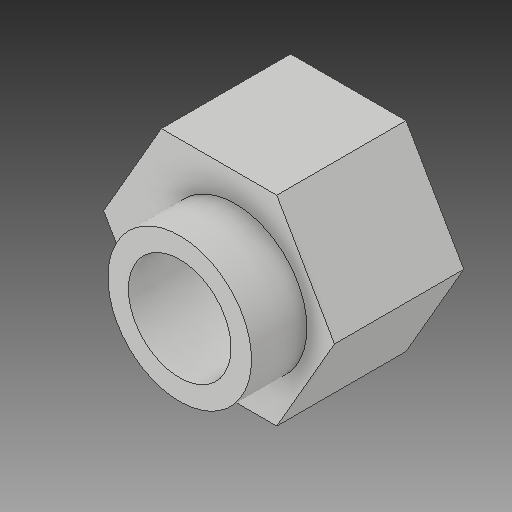
# Autodesk Inventor part: Eccentric Spacer
Saved by Autodesk Inventor 2018 (Build 220112000, 112)
## iProperties
Created: 2016-07-20
Part Number: Eccentric Spacer
Material: Generic
Document SubType Name: Modeling
Designer: User
Density: 1 g/cm^3
Appearance: Default
Mass: 0.445084 g
Surface Area: 5.38512 cm^2
Volume: 0.445084 cm^3
Author: User
Autodesk Inventor part; units mm, degrees
ref_plane "YZ Plane" through (0, 0, 0) normal (1, 0, 0) x (0, 1, 0)
ref_plane "XZ Plane" through (0, 0, 0) normal (0, 1, 0) x (-1, 0, 0)
ref_plane "XY Plane" through (0, 0, 0) normal (0, 0, 1) x (1, 0, 0)
sketch "Sketch1" plane through (0, 0, 0) normal (0, 0, 1) x (1, 0, 0)
  line L0 (-3.5818, 0) -> (-9.2068, 0)
  line L1 (-9.2068, 0) -> (-6.3943, 4.8714)
  line L2 (-6.3943, 4.8714) -> (-0.7693, 4.8714)
  line L3 (-0.7693, 4.8714) -> (2.0432, 0)
  line L4 (2.0432, 0) -> (-0.7693, -4.8714)
  line L5 (-0.7693, -4.8714) -> (-6.3943, -4.8714)
  line L6 (-6.3943, -4.8714) -> (-9.2068, 0)
  point P0 (-0.7818, 0)
  dimension "d0" = 5.625
  constraints: 14 end point, 1 coincident, 13 other
  measures "d0" distance of L0.start L0.end
extrude "Extrusion1" add sketch "Sketch1" along normal blind 6.3
sketch "Sketch2" plane through (0, 0, 6.3) normal (0, 0, 1) x (1, 0, 0)
  circle A0 centre (-2.8, 0) radius 2.5 projected
  circle A1 centre (-2.8, 0) radius 3.5
  point P0 (0, 0)
  dimension "d3" = 7
  constraints: 1 centre point, 1 coincident
  measures "d3" diameter of A1
extrude "Extrusion2" add sketch "Sketch2" along normal blind 2.7
sketch "Sketch3" plane through (-2.8, 0, 6.3) normal (0, 0, 1) x (1, 0, 0)
  circle A0 centre (0, 0) radius 2.5 projected
  point P0 (2.8, 0)
extrude "Extrusion3" cut sketch "Sketch3" against normal through all
body "Solid1"
